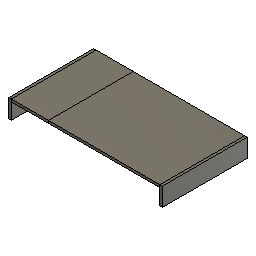
capstone final CAD (Autodesk Fusion 360 design; units mm, degrees)
Autodesk Fusion 360 part; units mm, degrees
sketch "Sketch1" plane through (0, 0, 0) normal (0, 1, 0) x (1, 0, 0)
  line L0 (88.9, -203.2) -> (-88.9, -203.2)
  line L1 (-88.9, -203.2) -> (-88.9, 203.2)
  line L2 (-88.9, 203.2) -> (88.9, 203.2)
  line L3 (88.9, 203.2) -> (88.9, -203.2)
  line L4 (88.9, -203.2) -> (-88.9, 203.2) construction
  line L5 (-88.9, -203.2) -> (88.9, 203.2) construction
  dimension "d1" = 406.4
  dimension "d2" = 177.8
  constraint horizontal L0
  constraint perpendicular L0 L1
  constraint parallel L0 L2
  constraint parallel L1 L3
  constraint coincident L4 origin
  constraint coincident L5 origin
  measures "d1" distance of L0.end L1.end
  measures "d2" distance of L1 L3
extrude "Extrude1" add sketch "Sketch1" along normal blind 12 makes body 1
extrude "Extrude2" add 1 faces at (88.9, 4, -67.7333) along direction (1, 0, 0) blind 533.4 separate body on bodies 1 makes body 2
sketch "Sketch2" plane through (0, 0, 0) normal (1, 0, 0) x (0, 0, -1)
  line L0 (203.5936, 11.7412, -90) -> (-202.8064, 11.7412, -90)
  line L1 (-202.8064, 11.7412, -90) -> (-202.8064, -64.4588, -90)
  line L2 (-202.8064, -64.4588, -90) -> (203.5936, -64.4588, -90)
  line L3 (203.5936, -64.4588, -90) -> (203.5936, 11.7412, -90)
  dimension "d7" = 406.4
  dimension "d8" = 76.2
extrude "Extrude3" add sketch "Sketch2" against normal blind 12 separate body contours L0 L1 L2 L3 in plane through (-90, 0, 0) normal (1, 0, 0) makes body 3
sketch "Sketch3" plane through (-88.9, 0, 0) normal (-1, 0, 0) x (0, 0, 1)
  line L0 (-203.2, 0) -> (203.2, 0)
  line L1 (203.2, 0) -> (203.2, 12)
  line L2 (203.2, 12) -> (-203.2, 12)
  line L3 (-203.2, 12) -> (-203.2, 0)
  line L4 (-203.2, 12) -> (203.2, 12)
  line L5 (203.2, 12) -> (203.2, 0)
  line L6 (203.2, 0) -> (-203.2, 0)
  line L7 (-203.2, 0) -> (-203.2, 12)
  constraint horizontal L4
  constraint vertical L5
  constraint horizontal L6
  constraint vertical L7
  constraint coincident L0.end L1.start
  constraint coincident L2.end L3.start
extrude "Extrude4" add sketch "Sketch3" along normal blind 12 separate body makes body 4
move_face "OffsetFaces1" offset 76.2 1 faces at (-92.9, 0, -67.7333) on bodies 4
ref_plane "WorkPlane1" through (266.7, 6, 0) normal (1, 0, 0) x (0, 0, -1)
mirror "Mirror1" about plane through (266.7, 6, 0) normal (1, 0, 0) of bodies 4 makes body 5
hidden bodies 3
